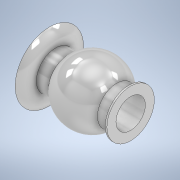
# Autodesk Inventor part: Bola grande
Saved by Autodesk Inventor 2020 (Build 240168000, 168)
## iProperties
Created: 2019-09-26
Part Number: Bola grande
Material: Aluminio 6061
Document SubType Name: Modeling
Designer: Frederich Schnëider
Density: 2.7 g/cm^3
Appearance: Aluminio - Pulido
Author: Frederich Schnëider
Autodesk Inventor part; units mm, degrees
sketch "Boceto1" plane through (0, 0, 0) normal (0, 0, 1) x (1, 0, 0)
  arc A0 (0, -2.75) -> (0, 2.75) centre (0, 0) ccw
  line L0 (0, 2.75) -> (0, -2.75)
  dimension "d0" = 5.5
  constraints: 2 end point, 2 point on circle, 1 centre point, 1 coincident, 1 vertical
  measures "d0" diameter of A0
revolve "Revolución1" add sketch "Boceto1" angle 360 about axis through (0, 2.75, 0) along (0, -1, 0)
ref_plane "Plano de trabajo2" through (2.75, 0, 0) normal (1, 0, 0) x (0, 1, 0)
ref_plane "Plano de trabajo3" through (-2.75, 0, 0) normal (1, 0, 0) x (0, 1, 0)
sketch "Boceto7" plane through (2.75, 0, 0) normal (1, 0, 0) x (0, 1, 0)
  circle A0 centre (0, 0) radius 1.7
  circle A1 centre (0, 0) radius 1.3
  dimension "d21" = 3.4
  dimension "d22" = 0.4
  constraints: 2 centre point, 1 coincident
  measures "d21" diameter of A0
  measures "d22" radial gap between concentric circles of A0 A1
extrude "Extrusión5" add sketch "Boceto7" along normal blind 0.5 and the other way blind 1
sketch "Boceto8" plane through (-2.75, 0, 0) normal (1, 0, 0) x (0, 1, 0)
  circle A0 centre (0, 0) radius 1.7
  circle A1 centre (0, 0) radius 1.7 projected
  circle A2 centre (0, 0) radius 1.3
  dimension "d27" = 3.4
  dimension "d35" = 2.6
  constraints: 2 centre point, 2 coincident
  measures "d27" diameter of A0
  measures "d35" diameter of A2
extrude "Extrusión6" add sketch "Boceto8" along normal blind 1 and the other way blind 0.5 contours A0 | A2
ref_plane "Plano de trabajo6" through (2.75, 0, 0) normal (1, 0, 0) x (0, 1, 0)
sketch "Boceto10" plane through (2.75, 0, 0) normal (1, 0, 0) x (0, 1, 0)
  circle A0 centre (0, 0) radius 1.3 projected
extrude "Extrusión8" cut sketch "Boceto10" against normal blind 10
ref_plane "Plano de trabajo7" through (3.25, 0, 0) normal (1, 0, 0) x (0, 0, -1)
sketch "Boceto11" plane through (3.25, 0, 0) normal (1, 0, 0) x (0, 0, -1)
  circle A0 centre (0, 0) radius 2.1
  circle A1 centre (0, 0) radius 1.3 projected
  dimension "d39" = 4.2
  constraints: 1 centre point, 1 coincident
  measures "d39" diameter of A0
extrude "Extrusión9" add sketch "Boceto11" along normal blind 0.15
ref_plane "Plano de trabajo9" through (-3.7, 0, 0) normal (-1, 0, 0) x (0, 0, 1)
ref_plane "Plano de trabajo8" through (-3.25, 0, 0) normal (-1, 0, 0) x (0, 0, 1)
sketch "Boceto12" plane through (-3.7, 0, 0) normal (-1, 0, 0) x (0, 0, 1)
  circle A0 centre (0, 0) radius 3.03
  circle A1 centre (0, 0) radius 1.3 projected
  dimension "d44" = 6.06
  constraints: 1 centre point, 1 coincident
  measures "d44" diameter of A0
extrude "Extrusión10" add sketch "Boceto12" along normal blind 0.1 and the other way blind 0.45
fillet "Empalme1" radius 2 1 edges at (-3.25, 0, -3.03)
